Autodesk Fusion 360 part; units mm, degrees
(part 24 of 40)
  line L3969 (68.5452, -19.8469) -> (68.5908, -19.8966) construction
  line L3970 (68.5908, -19.8966) -> (68.6136, -19.9215) construction
  line L3971 (-51.1066, 30.2798) -> (-52.5103, 31.1115)
  line L3972 (54.5366, 23.5481) -> (56.0345, 24.1948)
  line L3973 (57.9623, 13.005) -> (59.5542, 13.3622)
  line L3974 (13.005, -57.9623) -> (13.3622, -59.5542)
  arc A98 (67.2191, -24.2132) -> (68.6136, -19.9215) centre (0, 0) ccw
  line L3975 (30.2798, 51.1066) -> (31.1115, 52.5103)
  spline S53 degree 5 poles (45.8153, 40.3263) (45.8385, 40.3467) (45.8854, 40.3868) (45.9573, 40.4451) (46.056, 40.5192) (46.1833, 40.6066) (46.3135, 40.6904) (46.4454, 40.772) (46.5782, 40.8524) (46.7117, 40.932) (46.8458, 41.0107) (46.9807, 41.0883) (47.1168, 41.1642) (47.2543, 41.2383) (47.393, 41.3106) (47.5329, 41.3813) (47.6738, 41.4504) (47.8156, 41.5184) (47.9581, 41.5853) (48.1012, 41.6512) (48.245, 41.716) (48.3895, 41.7798) (48.5347, 41.8424) (48.6807, 41.9039) (48.8274, 41.9642) (48.9749, 42.0234) (49.123, 42.0815) (49.2717, 42.1386) (49.421, 42.1947) (49.5709, 42.2499) (49.7214, 42.3041) (49.8724, 42.3574) (50.024, 42.4097) (50.1761, 42.461) (50.3288, 42.5114) (50.482, 42.5608) (50.6358, 42.6094) (50.79, 42.657) (50.9447, 42.7037) (51.0999, 42.7495) (51.2556, 42.7945) (51.4118, 42.8386) (51.5684, 42.8818) (51.7255, 42.9241) (51.883, 42.9656) (52.0409, 43.0063) (52.1993, 43.0461) (52.3581, 43.085) (52.5173, 43.1231) (52.6769, 43.1604) (52.8369, 43.1969) (52.9973, 43.2326) (53.1581, 43.2674) (53.3193, 43.3015) (53.4809, 43.3347) (53.6428, 43.3672) (53.8051, 43.3988) (53.9677, 43.4297) (54.1307, 43.4597) (54.294, 43.489) (54.4577, 43.5175) (54.6217, 43.5453) (54.7861, 43.5723) (54.9508, 43.5984) (55.1158, 43.6239) (55.2811, 43.6486) (55.4467, 43.6725) (55.6126, 43.6956) (55.7789, 43.718) (55.9454, 43.7397) (56.1122, 43.7606) (56.2459, 43.7767) (56.3463, 43.7885) (56.4133, 43.7962) (56.4469, 43.8) knots 0 0 0 0 0 0 0.01428571 0.02857143 0.04285714 0.05714286 0.07142857 0.08571429 0.1 0.11428571 0.12857143 0.14285714 0.15714286 0.17142857 0.18571429 0.2 0.21428571 0.22857143 0.24285714 0.25714286 0.27142857 0.28571429 0.3 0.31428571 0.32857143 0.34285714 0.35714286 0.37142857 0.38571429 0.4 0.41428571 0.42857143 0.44285714 0.45714286 0.47142857 0.48571429 0.5 0.51428571 0.52857143 0.54285714 0.55714286 0.57142857 0.58571429 0.6 0.61428571 0.62857143 0.64285714 0.65714286 0.67142857 0.68571429 0.7 0.71428571 0.72857143 0.74285714 0.75714286 0.77142857 0.78571429 0.8 0.81428571 0.82857143 0.84285714 0.85714286 0.87142857 0.88571429 0.9 0.91428571 0.92857143 0.94285714 0.95714286 0.97142857 0.98571429 1 1 1 1 1 1
  line L3976 (45.8153, 40.3263) -> (45.8385, 40.3467) construction
  line L3977 (45.8385, 40.3467) -> (45.8854, 40.3868) construction
  line L3978 (45.8854, 40.3868) -> (45.9573, 40.4451) construction
  line L3979 (45.9573, 40.4451) -> (46.056, 40.5192) construction
  line L3980 (46.056, 40.5192) -> (46.1833, 40.6066) construction
  line L3981 (46.1833, 40.6066) -> (46.3135, 40.6904) construction
  line L3982 (46.3135, 40.6904) -> (46.4454, 40.772) construction
  line L3983 (46.4454, 40.772) -> (46.5782, 40.8524) construction
  line L3984 (46.5782, 40.8524) -> (46.7117, 40.932) construction
  line L3985 (46.7117, 40.932) -> (46.8458, 41.0107) construction
  line L3986 (46.8458, 41.0107) -> (46.9807, 41.0883) construction
  line L3987 (46.9807, 41.0883) -> (47.1168, 41.1642) construction
  line L3988 (47.1168, 41.1642) -> (47.2543, 41.2383) construction
  line L3989 (47.2543, 41.2383) -> (47.393, 41.3106) construction
  line L3990 (47.393, 41.3106) -> (47.5329, 41.3813) construction
  line L3991 (47.5329, 41.3813) -> (47.6738, 41.4504) construction
  line L3992 (47.6738, 41.4504) -> (47.8156, 41.5184) construction
  line L3993 (47.8156, 41.5184) -> (47.9581, 41.5853) construction
  line L3994 (47.9581, 41.5853) -> (48.1012, 41.6512) construction
  line L3995 (48.1012, 41.6512) -> (48.245, 41.716) construction
  line L3996 (48.245, 41.716) -> (48.3895, 41.7798) construction
  line L3997 (48.3895, 41.7798) -> (48.5347, 41.8424) construction
  line L3998 (48.5347, 41.8424) -> (48.6807, 41.9039) construction
  line L3999 (48.6807, 41.9039) -> (48.8274, 41.9642) construction
  line L4000 (48.8274, 41.9642) -> (48.9749, 42.0234) construction
  line L4001 (48.9749, 42.0234) -> (49.123, 42.0815) construction
  line L4002 (49.123, 42.0815) -> (49.2717, 42.1386) construction
  line L4003 (49.2717, 42.1386) -> (49.421, 42.1947) construction
  line L4004 (49.421, 42.1947) -> (49.5709, 42.2499) construction
  line L4005 (49.5709, 42.2499) -> (49.7214, 42.3041) construction
  line L4006 (49.7214, 42.3041) -> (49.8724, 42.3574) construction
  line L4007 (49.8724, 42.3574) -> (50.024, 42.4097) construction
  line L4008 (50.024, 42.4097) -> (50.1761, 42.461) construction
  line L4009 (50.1761, 42.461) -> (50.3288, 42.5114) construction
  line L4010 (50.3288, 42.5114) -> (50.482, 42.5608) construction
  line L4011 (50.482, 42.5608) -> (50.6358, 42.6094) construction
  line L4012 (50.6358, 42.6094) -> (50.79, 42.657) construction
  line L4013 (50.79, 42.657) -> (50.9447, 42.7037) construction
  line L4014 (50.9447, 42.7037) -> (51.0999, 42.7495) construction
  line L4015 (51.0999, 42.7495) -> (51.2556, 42.7945) construction
  line L4016 (51.2556, 42.7945) -> (51.4118, 42.8386) construction
  line L4017 (51.4118, 42.8386) -> (51.5684, 42.8818) construction
  line L4018 (51.5684, 42.8818) -> (51.7255, 42.9241) construction
  line L4019 (51.7255, 42.9241) -> (51.883, 42.9656) construction
  line L4020 (51.883, 42.9656) -> (52.0409, 43.0063) construction
  line L4021 (52.0409, 43.0063) -> (52.1993, 43.0461) construction
  line L4022 (52.1993, 43.0461) -> (52.3581, 43.085) construction
  line L4023 (52.3581, 43.085) -> (52.5173, 43.1231) construction
  line L4024 (52.5173, 43.1231) -> (52.6769, 43.1604) construction
  line L4025 (52.6769, 43.1604) -> (52.8369, 43.1969) construction
  line L4026 (52.8369, 43.1969) -> (52.9973, 43.2326) construction
  line L4027 (52.9973, 43.2326) -> (53.1581, 43.2674) construction
  line L4028 (53.1581, 43.2674) -> (53.3193, 43.3015) construction
  line L4029 (53.3193, 43.3015) -> (53.4809, 43.3347) construction
  line L4030 (53.4809, 43.3347) -> (53.6428, 43.3672) construction
  line L4031 (53.6428, 43.3672) -> (53.8051, 43.3988) construction
  line L4032 (53.8051, 43.3988) -> (53.9677, 43.4297) construction
  line L4033 (53.9677, 43.4297) -> (54.1307, 43.4597) construction
  line L4034 (54.1307, 43.4597) -> (54.294, 43.489) construction
  line L4035 (54.294, 43.489) -> (54.4577, 43.5175) construction
  line L4036 (54.4577, 43.5175) -> (54.6217, 43.5453) construction
  line L4037 (54.6217, 43.5453) -> (54.7861, 43.5723) construction
  line L4038 (54.7861, 43.5723) -> (54.9508, 43.5984) construction
  line L4039 (54.9508, 43.5984) -> (55.1158, 43.6239) construction
  line L4040 (55.1158, 43.6239) -> (55.2811, 43.6486) construction
  line L4041 (55.2811, 43.6486) -> (55.4467, 43.6725) construction
  line L4042 (55.4467, 43.6725) -> (55.6126, 43.6956) construction
  line L4043 (55.6126, 43.6956) -> (55.7789, 43.718) construction
  line L4044 (55.7789, 43.718) -> (55.9454, 43.7397) construction
  line L4045 (55.9454, 43.7397) -> (56.1122, 43.7606) construction
  line L4046 (56.1122, 43.7606) -> (56.2459, 43.7767) construction
  line L4047 (56.2459, 43.7767) -> (56.3463, 43.7885) construction
  line L4048 (56.3463, 43.7885) -> (56.4133, 43.7962) construction
  line L4049 (56.4133, 43.7962) -> (56.4469, 43.8) construction
  arc A99 (7.2806, -56.9737) -> (5.5428, -59.1442) centre (7.5341, -58.9575) ccw
  arc A100 (27.5982, 50.3721) -> (24.5301, 51.9354) centre (0, 0) ccw
  arc A101 (-56.9737, -7.2806) -> (-59.1442, -5.5428) centre (-58.9575, -7.5341) ccw
  arc A102 (51.1066, 30.2798) -> (50.3721, 27.5982) centre (52.1261, 28.5592) ccw
  arc A103 (7.2806, -56.9737) -> (10.6816, -56.435) centre (0, 0) ccw
  arc A104 (-44.5906, 39.2483) -> (-41.8132, 39.3784) centre (-43.2692, 40.7496) ccw
  spline S54 degree 5 poles (-5.6951, -60.7685) (-5.6979, -60.7993) (-5.7029, -60.8609) (-5.7078, -60.9533) (-5.7097, -61.0766) (-5.7056, -61.231) (-5.6969, -61.3856) (-5.6854, -61.5403) (-5.6723, -61.695) (-5.6583, -61.8498) (-5.6431, -62.0045) (-5.6265, -62.1593) (-5.608, -62.314) (-5.5871, -62.4688) (-5.5641, -62.6235) (-5.539, -62.7782) (-5.5121, -62.9329) (-5.4838, -63.0875) (-5.4542, -63.2421) (-5.4233, -63.3966) (-5.3913, -63.5511) (-5.3579, -63.7055) (-5.3232, -63.8598) (-5.2871, -64.014) (-5.2497, -64.1682) (-5.2109, -64.3222) (-5.1709, -64.4762) (-5.1297, -64.6301) (-5.0873, -64.7839) (-5.0439, -64.9376) (-4.9993, -65.0912) (-4.9536, -65.2447) (-4.9068, -65.398) (-4.8589, -65.5513) (-4.8099, -65.7044) (-4.7599, -65.8574) (-4.7087, -66.0103) (-4.6566, -66.1631) (-4.6035, -66.3158) (-4.5493, -66.4683) (-4.4942, -66.6206) (-4.438, -66.7729) (-4.381, -66.925) (-4.3229, -67.077) (-4.2639, -67.2288) (-4.2039, -67.3804) (-4.143, -67.532) (-4.0812, -67.6833) (-4.0185, -67.8345) (-3.9548, -67.9856) (-3.8903, -68.1365) (-3.8249, -68.2872) (-3.7585, -68.4378) (-3.6913, -68.5882) (-3.6233, -68.7384) (-3.5543, -68.8885) (-3.4846, -69.0384) (-3.4139, -69.1881) (-3.3425, -69.3376) (-3.2701, -69.487) (-3.197, -69.6362) (-3.123, -69.7852) (-3.0482, -69.934) (-2.9726, -70.0826) (-2.8962, -70.2311) (-2.819, -70.3793) (-2.741, -70.5274) (-2.6622, -70.6752) (-2.5826, -70.8229) (-2.5023, -70.9703) (-2.4211, -71.1176) (-2.3556, -71.2352) (-2.3061, -71.3234) (-2.2729, -71.3821) (-2.2563, -71.4115) knots 0 0 0 0 0 0 0.01428571 0.02857143 0.04285714 0.05714286 0.07142857 0.08571429 0.1 0.11428571 0.12857143 0.14285714 0.15714286 0.17142857 0.18571429 0.2 0.21428571 0.22857143 0.24285714 0.25714286 0.27142857 0.28571429 0.3 0.31428571 0.32857143 0.34285714 0.35714286 0.37142857 0.38571429 0.4 0.41428571 0.42857143 0.44285714 0.45714286 0.47142857 0.48571429 0.5 0.51428571 0.52857143 0.54285714 0.55714286 0.57142857 0.58571429 0.6 0.61428571 0.62857143 0.64285714 0.65714286 0.67142857 0.68571429 0.7 0.71428571 0.72857143 0.74285714 0.75714286 0.77142857 0.78571429 0.8 0.81428571 0.82857143 0.84285714 0.85714286 0.87142857 0.88571429 0.9 0.91428571 0.92857143 0.94285714 0.95714286 0.97142857 0.98571429 1 1 1 1 1 1
  line L4050 (-5.6951, -60.7685) -> (-5.6979, -60.7993) construction
  line L4051 (-5.6979, -60.7993) -> (-5.7029, -60.8609) construction
  line L4052 (-5.7029, -60.8609) -> (-5.7078, -60.9533) construction
  line L4053 (-5.7078, -60.9533) -> (-5.7097, -61.0766) construction
  line L4054 (-5.7097, -61.0766) -> (-5.7056, -61.231) construction
  line L4055 (-5.7056, -61.231) -> (-5.6969, -61.3856) construction
  line L4056 (-5.6969, -61.3856) -> (-5.6854, -61.5403) construction
  line L4057 (-5.6854, -61.5403) -> (-5.6723, -61.695) construction
  line L4058 (-5.6723, -61.695) -> (-5.6583, -61.8498) construction
  line L4059 (-5.6583, -61.8498) -> (-5.6431, -62.0045) construction
  line L4060 (-5.6431, -62.0045) -> (-5.6265, -62.1593) construction
  line L4061 (-5.6265, -62.1593) -> (-5.608, -62.314) construction
  line L4062 (-5.608, -62.314) -> (-5.5871, -62.4688) construction
  line L4063 (-5.5871, -62.4688) -> (-5.5641, -62.6235) construction
  line L4064 (-5.5641, -62.6235) -> (-5.539, -62.7782) construction
  line L4065 (-5.539, -62.7782) -> (-5.5121, -62.9329) construction
  line L4066 (-5.5121, -62.9329) -> (-5.4838, -63.0875) construction
  line L4067 (-5.4838, -63.0875) -> (-5.4542, -63.2421) construction
  line L4068 (-5.4542, -63.2421) -> (-5.4233, -63.3966) construction
  line L4069 (-5.4233, -63.3966) -> (-5.3913, -63.5511) construction
  line L4070 (-5.3913, -63.5511) -> (-5.3579, -63.7055) construction
  line L4071 (-5.3579, -63.7055) -> (-5.3232, -63.8598) construction
  line L4072 (-5.3232, -63.8598) -> (-5.2871, -64.014) construction
  line L4073 (-5.2871, -64.014) -> (-5.2497, -64.1682) construction
  line L4074 (-5.2497, -64.1682) -> (-5.2109, -64.3222) construction
  line L4075 (-5.2109, -64.3222) -> (-5.1709, -64.4762) construction
  line L4076 (-5.1709, -64.4762) -> (-5.1297, -64.6301) construction
  line L4077 (-5.1297, -64.6301) -> (-5.0873, -64.7839) construction
  line L4078 (-5.0873, -64.7839) -> (-5.0439, -64.9376) construction
  line L4079 (-5.0439, -64.9376) -> (-4.9993, -65.0912) construction
  line L4080 (-4.9993, -65.0912) -> (-4.9536, -65.2447) construction
  line L4081 (-4.9536, -65.2447) -> (-4.9068, -65.398) construction
  line L4082 (-4.9068, -65.398) -> (-4.8589, -65.5513) construction
  line L4083 (-4.8589, -65.5513) -> (-4.8099, -65.7044) construction
  line L4084 (-4.8099, -65.7044) -> (-4.7599, -65.8574) construction
  line L4085 (-4.7599, -65.8574) -> (-4.7087, -66.0103) construction
  line L4086 (-4.7087, -66.0103) -> (-4.6566, -66.1631) construction
  line L4087 (-4.6566, -66.1631) -> (-4.6035, -66.3158) construction
  line L4088 (-4.6035, -66.3158) -> (-4.5493, -66.4683) construction
  line L4089 (-4.5493, -66.4683) -> (-4.4942, -66.6206) construction
  line L4090 (-4.4942, -66.6206) -> (-4.438, -66.7729) construction
  line L4091 (-4.438, -66.7729) -> (-4.381, -66.925) construction
  line L4092 (-4.381, -66.925) -> (-4.3229, -67.077) construction
  line L4093 (-4.3229, -67.077) -> (-4.2639, -67.2288) construction
  line L4094 (-4.2639, -67.2288) -> (-4.2039, -67.3804) construction
  line L4095 (-4.2039, -67.3804) -> (-4.143, -67.532) construction
  line L4096 (-4.143, -67.532) -> (-4.0812, -67.6833) construction
  line L4097 (-4.0812, -67.6833) -> (-4.0185, -67.8345) construction
  line L4098 (-4.0185, -67.8345) -> (-3.9548, -67.9856) construction
  line L4099 (-3.9548, -67.9856) -> (-3.8903, -68.1365) construction
  line L4100 (-3.8903, -68.1365) -> (-3.8249, -68.2872) construction
  line L4101 (-3.8249, -68.2872) -> (-3.7585, -68.4378) construction
  line L4102 (-3.7585, -68.4378) -> (-3.6913, -68.5882) construction
  line L4103 (-3.6913, -68.5882) -> (-3.6233, -68.7384) construction
  line L4104 (-3.6233, -68.7384) -> (-3.5543, -68.8885) construction
  line L4105 (-3.5543, -68.8885) -> (-3.4846, -69.0384) construction
  line L4106 (-3.4846, -69.0384) -> (-3.4139, -69.1881) construction
  line L4107 (-3.4139, -69.1881) -> (-3.3425, -69.3376) construction
  line L4108 (-3.3425, -69.3376) -> (-3.2701, -69.487) construction
  line L4109 (-3.2701, -69.487) -> (-3.197, -69.6362) construction
  line L4110 (-3.197, -69.6362) -> (-3.123, -69.7852) construction
  line L4111 (-3.123, -69.7852) -> (-3.0482, -69.934) construction
  line L4112 (-3.0482, -69.934) -> (-2.9726, -70.0826) construction
  line L4113 (-2.9726, -70.0826) -> (-2.8962, -70.2311) construction
  line L4114 (-2.8962, -70.2311) -> (-2.819, -70.3793) construction
  line L4115 (-2.819, -70.3793) -> (-2.741, -70.5274) construction
  line L4116 (-2.741, -70.5274) -> (-2.6622, -70.6752) construction
  line L4117 (-2.6622, -70.6752) -> (-2.5826, -70.8229) construction
  line L4118 (-2.5826, -70.8229) -> (-2.5023, -70.9703) construction
  line L4119 (-2.5023, -70.9703) -> (-2.4211, -71.1176) construction
  line L4120 (-2.4211, -71.1176) -> (-2.3556, -71.2352) construction
  line L4121 (-2.3556, -71.2352) -> (-2.3061, -71.3234) construction
  line L4122 (-2.3061, -71.3234) -> (-2.2729, -71.3821) construction
  line L4123 (-2.2729, -71.3821) -> (-2.2563, -71.4115) construction
  spline S55 degree 5 poles (31.1115, -52.5103) (31.1272, -52.5368) (31.1594, -52.5895) (31.2097, -52.6672) (31.2807, -52.7681) (31.3748, -52.8906) (31.4727, -53.0106) (31.5729, -53.1289) (31.6744, -53.2464) (31.7767, -53.3634) (31.88, -53.4797) (31.9844, -53.5951) (32.0903, -53.7094) (32.1981, -53.8224) (32.3077, -53.934) (32.419, -54.0444) (32.5316, -54.1537) (32.6455, -54.2622) (32.7603, -54.3698) (32.876, -54.4767) (32.9927, -54.5828) (33.1105, -54.6881) (33.2292, -54.7926) (33.3491, -54.8961) (33.47, -54.9988) (33.5919, -55.1007) (33.7148, -55.2017) (33.8386, -55.302) (33.9633, -55.4015) (34.0888, -55.5003) (34.2151, -55.5984) (34.3423, -55.6957) (34.4703, -55.7923) (34.5991, -55.8881) (34.7288, -55.9832) (34.8592, -56.0776) (34.9905, -56.1712) (35.1224, -56.2642) (35.2552, -56.3564) (35.3886, -56.448) (35.5228, -56.5388) (35.6577, -56.629) (35.7933, -56.7185) (35.9295, -56.8073) (36.0665, -56.8955) (36.2042, -56.9829) (36.3425, -57.0697) (36.4815, -57.1558) (36.6211, -57.2413) (36.7614, -57.3261) (36.9023, -57.4102) (37.0438, -57.4937) (37.186, -57.5765) (37.3288, -57.6587) (37.4721, -57.7403) (37.6161, -57.8212) (37.7607, -57.9014) (37.9058, -57.981) (38.0515, -58.06) (38.1978, -58.1383) (38.3447, -58.216) (38.4921, -58.2931) (38.6401, -58.3695) (38.7886, -58.4453) (38.9377, -58.5205) (39.0873, -58.595) (39.2374, -58.669) (39.3881, -58.7423) (39.5393, -58.8149) (39.6909, -58.887) (39.8431, -58.9584) (39.9653, -59.0151) (40.0572, -59.0573) (40.1185, -59.0853) (40.1492, -59.0993) knots 0 0 0 0 0 0 0.01428571 0.02857143 0.04285714 0.05714286 0.07142857 0.08571429 0.1 0.11428571 0.12857143 0.14285714 0.15714286 0.17142857 0.18571429 0.2 0.21428571 0.22857143 0.24285714 0.25714286 0.27142857 0.28571429 0.3 0.31428571 0.32857143 0.34285714 0.35714286 0.37142857 0.38571429 0.4 0.41428571 0.42857143 0.44285714 0.45714286 0.47142857 0.48571429 0.5 0.51428571 0.52857143 0.54285714 0.55714286 0.57142857 0.58571429 0.6 0.61428571 0.62857143 0.64285714 0.65714286 0.67142857 0.68571429 0.7 0.71428571 0.72857143 0.74285714 0.75714286 0.77142857 0.78571429 0.8 0.81428571 0.82857143 0.84285714 0.85714286 0.87142857 0.88571429 0.9 0.91428571 0.92857143 0.94285714 0.95714286 0.97142857 0.98571429 1 1 1 1 1 1
  line L4124 (31.1115, -52.5103) -> (31.1272, -52.5368) construction
  line L4125 (31.1272, -52.5368) -> (31.1594, -52.5895) construction
  line L4126 (31.1594, -52.5895) -> (31.2097, -52.6672) construction
  line L4127 (31.2097, -52.6672) -> (31.2807, -52.7681) construction
  line L4128 (31.2807, -52.7681) -> (31.3748, -52.8906) construction
  line L4129 (31.3748, -52.8906) -> (31.4727, -53.0106) construction
  line L4130 (31.4727, -53.0106) -> (31.5729, -53.1289) construction
  line L4131 (31.5729, -53.1289) -> (31.6744, -53.2464) construction
  line L4132 (31.6744, -53.2464) -> (31.7767, -53.3634) construction
  line L4133 (31.7767, -53.3634) -> (31.88, -53.4797) construction
  line L4134 (31.88, -53.4797) -> (31.9844, -53.5951) construction
  line L4135 (31.9844, -53.5951) -> (32.0903, -53.7094) construction
  line L4136 (32.0903, -53.7094) -> (32.1981, -53.8224) construction
  line L4137 (32.1981, -53.8224) -> (32.3077, -53.934) construction
  line L4138 (32.3077, -53.934) -> (32.419, -54.0444) construction
  line L4139 (32.419, -54.0444) -> (32.5316, -54.1537) construction
  line L4140 (32.5316, -54.1537) -> (32.6455, -54.2622) construction
  line L4141 (32.6455, -54.2622) -> (32.7603, -54.3698) construction
  line L4142 (32.7603, -54.3698) -> (32.876, -54.4767) construction
  line L4143 (32.876, -54.4767) -> (32.9927, -54.5828) construction
  line L4144 (32.9927, -54.5828) -> (33.1105, -54.6881) construction
  line L4145 (33.1105, -54.6881) -> (33.2292, -54.7926) construction
  line L4146 (33.2292, -54.7926) -> (33.3491, -54.8961) construction
  line L4147 (33.3491, -54.8961) -> (33.47, -54.9988) construction
  line L4148 (33.47, -54.9988) -> (33.5919, -55.1007) construction
  line L4149 (33.5919, -55.1007) -> (33.7148, -55.2017) construction
  line L4150 (33.7148, -55.2017) -> (33.8386, -55.302) construction
  line L4151 (33.8386, -55.302) -> (33.9633, -55.4015) construction
  line L4152 (33.9633, -55.4015) -> (34.0888, -55.5003) construction
  line L4153 (34.0888, -55.5003) -> (34.2151, -55.5984) construction
  line L4154 (34.2151, -55.5984) -> (34.3423, -55.6957) construction
  line L4155 (34.3423, -55.6957) -> (34.4703, -55.7923) construction
  line L4156 (34.4703, -55.7923) -> (34.5991, -55.8881) construction
  line L4157 (34.5991, -55.8881) -> (34.7288, -55.9832) construction
  line L4158 (34.7288, -55.9832) -> (34.8592, -56.0776) construction
  line L4159 (34.8592, -56.0776) -> (34.9905, -56.1712) construction
  line L4160 (34.9905, -56.1712) -> (35.1224, -56.2642) construction
  line L4161 (35.1224, -56.2642) -> (35.2552, -56.3564) construction
  line L4162 (35.2552, -56.3564) -> (35.3886, -56.448) construction
  line L4163 (35.3886, -56.448) -> (35.5228, -56.5388) construction
  line L4164 (35.5228, -56.5388) -> (35.6577, -56.629) construction
  line L4165 (35.6577, -56.629) -> (35.7933, -56.7185) construction
  line L4166 (35.7933, -56.7185) -> (35.9295, -56.8073) construction
  line L4167 (35.9295, -56.8073) -> (36.0665, -56.8955) construction
  line L4168 (36.0665, -56.8955) -> (36.2042, -56.9829) construction
  line L4169 (36.2042, -56.9829) -> (36.3425, -57.0697) construction
  line L4170 (36.3425, -57.0697) -> (36.4815, -57.1558) construction
  line L4171 (36.4815, -57.1558) -> (36.6211, -57.2413) construction
  line L4172 (36.6211, -57.2413) -> (36.7614, -57.3261) construction
  line L4173 (36.7614, -57.3261) -> (36.9023, -57.4102) construction
  line L4174 (36.9023, -57.4102) -> (37.0438, -57.4937) construction
  line L4175 (37.0438, -57.4937) -> (37.186, -57.5765) construction
  line L4176 (37.186, -57.5765) -> (37.3288, -57.6587) construction
  line L4177 (37.3288, -57.6587) -> (37.4721, -57.7403) construction
  line L4178 (37.4721, -57.7403) -> (37.6161, -57.8212) construction
  line L4179 (37.6161, -57.8212) -> (37.7607, -57.9014) construction
  line L4180 (37.7607, -57.9014) -> (37.9058, -57.981) construction
  line L4181 (37.9058, -57.981) -> (38.0515, -58.06) construction
  line L4182 (38.0515, -58.06) -> (38.1978, -58.1383) construction
  line L4183 (38.1978, -58.1383) -> (38.3447, -58.216) construction
  line L4184 (38.3447, -58.216) -> (38.4921, -58.2931) construction
  line L4185 (38.4921, -58.2931) -> (38.6401, -58.3695) construction
  line L4186 (38.6401, -58.3695) -> (38.7886, -58.4453) construction
  line L4187 (38.7886, -58.4453) -> (38.9377, -58.5205) construction
  line L4188 (38.9377, -58.5205) -> (39.0873, -58.595) construction
  line L4189 (39.0873, -58.595) -> (39.2374, -58.669) construction
  line L4190 (39.2374, -58.669) -> (39.3881, -58.7423) construction
  line L4191 (39.3881, -58.7423) -> (39.5393, -58.8149) construction
  line L4192 (39.5393, -58.8149) -> (39.6909, -58.887) construction
  line L4193 (39.6909, -58.887) -> (39.8431, -58.9584) construction
  line L4194 (39.8431, -58.9584) -> (39.9653, -59.0151) construction
  line L4195 (39.9653, -59.0151) -> (40.0572, -59.0573) construction
  line L4196 (40.0572, -59.0573) -> (40.1185, -59.0853) construction
  line L4197 (40.1185, -59.0853) -> (40.1492, -59.0993) construction
  line L4198 (-30.2798, -51.1066) -> (-31.1115, -52.5103)
  line L4199 (-39.2483, 44.5906) -> (-40.3263, 45.8153)
  arc A105 (-7.2806, 56.9737) -> (-5.5428, 59.1442) centre (-7.5341, 58.9575) ccw
  line L4200 (23.5481, -54.5366) -> (24.1948, -56.0345)
  arc A106 (56.9737, 7.2806) -> (56.435, 10.6816) centre (0, 0) ccw
  arc A107 (-10.6816, -56.435) -> (-7.2806, -56.9737) centre (0, 0) ccw
  spline S56 degree 5 poles (-13.3622, 59.5542) (-13.369, 59.5843) (-13.3833, 59.6444) (-13.4071, 59.7338) (-13.4435, 59.8517) (-13.4951, 59.9973) (-13.5511, 60.1416) (-13.6099, 60.2852) (-13.6701, 60.4283) (-13.7313, 60.5711) (-13.7935, 60.7136) (-13.8571, 60.8557) (-13.9226, 60.9971) (-13.9902, 61.1379) (-14.06, 61.2779) (-14.1316, 61.4173) (-14.205, 61.5561) (-14.2797, 61.6944) (-14.3557, 61.8322) (-14.4327, 61.9697) (-14.5109, 62.1067) (-14.5904, 62.2432) (-14.6711, 62.3792) (-14.753, 62.5148) (-14.8363, 62.6498) (-14.9208, 62.7843) (-15.0064, 62.9184) (-15.0932, 63.052) (-15.181, 63.1852) (-15.2698, 63.318) (-15.3597, 63.4503) (-15.4506, 63.5821) (-15.5425, 63.7135) (-15.6354, 63.8445) (-15.7293, 63.975) (-15.8242, 64.105) (-15.92, 64.2346) (-16.0168, 64.3638) (-16.1146, 64.4926) (-16.2132, 64.6209) (-16.3127, 64.7488) (-16.4131, 64.8762) (-16.5144, 65.0032) (-16.6166, 65.1298) (-16.7196, 65.256) (-16.8235, 65.3817) (-16.9283, 65.507) (-17.0338, 65.6318) (-17.1402, 65.7562) (-17.2474, 65.8802) (-17.3555, 66.0038) (-17.4643, 66.1269) (-17.5739, 66.2497) (-17.6842, 66.3719) (-17.7954, 66.4938) (-17.9073, 66.6152) (-18.02, 66.7362) (-18.1335, 66.8568) (-18.2477, 66.9769) (-18.3626, 67.0966) (-18.4782, 67.2159) (-18.5946, 67.3347) (-18.7118, 67.4531) (-18.8296, 67.5711) (-18.9481, 67.6887) (-19.0674, 67.8058) (-19.1873, 67.9225) (-19.3079, 68.0388) (-19.4293, 68.1546) (-19.5512, 68.27) (-19.6739, 68.385) (-19.7726, 68.4767) (-19.8469, 68.5452) (-19.8966, 68.5908) (-19.9215, 68.6136) knots 0 0 0 0 0 0 0.01428571 0.02857143 0.04285714 0.05714286 0.07142857 0.08571429 0.1 0.11428571 0.12857143 0.14285714 0.15714286 0.17142857 0.18571429 0.2 0.21428571 0.22857143 0.24285714 0.25714286 0.27142857 0.28571429 0.3 0.31428571 0.32857143 0.34285714 0.35714286 0.37142857 0.38571429 0.4 0.41428571 0.42857143 0.44285714 0.45714286 0.47142857 0.48571429 0.5 0.51428571 0.52857143 0.54285714 0.55714286 0.57142857 0.58571429 0.6 0.61428571 0.62857143 0.64285714 0.65714286 0.67142857 0.68571429 0.7 0.71428571 0.72857143 0.74285714 0.75714286 0.77142857 0.78571429 0.8 0.81428571 0.82857143 0.84285714 0.85714286 0.87142857 0.88571429 0.9 0.91428571 0.92857143 0.94285714 0.95714286 0.97142857 0.98571429 1 1 1 1 1 1
  line L4201 (-13.3622, 59.5542) -> (-13.369, 59.5843) construction
  line L4202 (-13.369, 59.5843) -> (-13.3833, 59.6444) construction
  line L4203 (-13.3833, 59.6444) -> (-13.4071, 59.7338) construction
  line L4204 (-13.4071, 59.7338) -> (-13.4435, 59.8517) construction
  line L4205 (-13.4435, 59.8517) -> (-13.4951, 59.9973) construction
  line L4206 (-13.4951, 59.9973) -> (-13.5511, 60.1416) construction
  line L4207 (-13.5511, 60.1416) -> (-13.6099, 60.2852) construction
  line L4208 (-13.6099, 60.2852) -> (-13.6701, 60.4283) construction
  line L4209 (-13.6701, 60.4283) -> (-13.7313, 60.5711) construction
  line L4210 (-13.7313, 60.5711) -> (-13.7935, 60.7136) construction
  line L4211 (-13.7935, 60.7136) -> (-13.8571, 60.8557) construction
  line L4212 (-13.8571, 60.8557) -> (-13.9226, 60.9971) construction
  line L4213 (-13.9226, 60.9971) -> (-13.9902, 61.1379) construction
  line L4214 (-13.9902, 61.1379) -> (-14.06, 61.2779) construction
  line L4215 (-14.06, 61.2779) -> (-14.1316, 61.4173) construction
  line L4216 (-14.1316, 61.4173) -> (-14.205, 61.5561) construction
  line L4217 (-14.205, 61.5561) -> (-14.2797, 61.6944) construction
  line L4218 (-14.2797, 61.6944) -> (-14.3557, 61.8322) construction
  line L4219 (-14.3557, 61.8322) -> (-14.4327, 61.9697) construction
  line L4220 (-14.4327, 61.9697) -> (-14.5109, 62.1067) construction
  line L4221 (-14.5109, 62.1067) -> (-14.5904, 62.2432) construction
  line L4222 (-14.5904, 62.2432) -> (-14.6711, 62.3792) construction
  line L4223 (-14.6711, 62.3792) -> (-14.753, 62.5148) construction
  line L4224 (-14.753, 62.5148) -> (-14.8363, 62.6498) construction
  line L4225 (-14.8363, 62.6498) -> (-14.9208, 62.7843) construction
  line L4226 (-14.9208, 62.7843) -> (-15.0064, 62.9184) construction
  line L4227 (-15.0064, 62.9184) -> (-15.0932, 63.052) construction
  line L4228 (-15.0932, 63.052) -> (-15.181, 63.1852) construction
  line L4229 (-15.181, 63.1852) -> (-15.2698, 63.318) construction
  line L4230 (-15.2698, 63.318) -> (-15.3597, 63.4503) construction
  line L4231 (-15.3597, 63.4503) -> (-15.4506, 63.5821) construction
  line L4232 (-15.4506, 63.5821) -> (-15.5425, 63.7135) construction
  line L4233 (-15.5425, 63.7135) -> (-15.6354, 63.8445) construction
  line L4234 (-15.6354, 63.8445) -> (-15.7293, 63.975) construction
  line L4235 (-15.7293, 63.975) -> (-15.8242, 64.105) construction
  line L4236 (-15.8242, 64.105) -> (-15.92, 64.2346) construction
  line L4237 (-15.92, 64.2346) -> (-16.0168, 64.3638) construction
  line L4238 (-16.0168, 64.3638) -> (-16.1146, 64.4926) construction
  line L4239 (-16.1146, 64.4926) -> (-16.2132, 64.6209) construction
  line L4240 (-16.2132, 64.6209) -> (-16.3127, 64.7488) construction
  line L4241 (-16.3127, 64.7488) -> (-16.4131, 64.8762) construction
  line L4242 (-16.4131, 64.8762) -> (-16.5144, 65.0032) construction
  line L4243 (-16.5144, 65.0032) -> (-16.6166, 65.1298) construction
  line L4244 (-16.6166, 65.1298) -> (-16.7196, 65.256) construction
  line L4245 (-16.7196, 65.256) -> (-16.8235, 65.3817) construction
  line L4246 (-16.8235, 65.3817) -> (-16.9283, 65.507) construction
  line L4247 (-16.9283, 65.507) -> (-17.0338, 65.6318) construction
  line L4248 (-17.0338, 65.6318) -> (-17.1402, 65.7562) construction
  line L4249 (-17.1402, 65.7562) -> (-17.2474, 65.8802) construction
  line L4250 (-17.2474, 65.8802) -> (-17.3555, 66.0038) construction
  line L4251 (-17.3555, 66.0038) -> (-17.4643, 66.1269) construction
  line L4252 (-17.4643, 66.1269) -> (-17.5739, 66.2497) construction
  line L4253 (-17.5739, 66.2497) -> (-17.6842, 66.3719) construction
  line L4254 (-17.6842, 66.3719) -> (-17.7954, 66.4938) construction
  line L4255 (-17.7954, 66.4938) -> (-17.9073, 66.6152) construction
  line L4256 (-17.9073, 66.6152) -> (-18.02, 66.7362) construction
  line L4257 (-18.02, 66.7362) -> (-18.1335, 66.8568) construction
  line L4258 (-18.1335, 66.8568) -> (-18.2477, 66.9769) construction
  line L4259 (-18.2477, 66.9769) -> (-18.3626, 67.0966) construction
  line L4260 (-18.3626, 67.0966) -> (-18.4782, 67.2159) construction
  line L4261 (-18.4782, 67.2159) -> (-18.5946, 67.3347) construction
  line L4262 (-18.5946, 67.3347) -> (-18.7118, 67.4531) construction
  line L4263 (-18.7118, 67.4531) -> (-18.8296, 67.5711) construction
  line L4264 (-18.8296, 67.5711) -> (-18.9481, 67.6887) construction
  line L4265 (-18.9481, 67.6887) -> (-19.0674, 67.8058) construction
  line L4266 (-19.0674, 67.8058) -> (-19.1873, 67.9225) construction
  line L4267 (-19.1873, 67.9225) -> (-19.3079, 68.0388) construction
  line L4268 (-19.3079, 68.0388) -> (-19.4293, 68.1546) construction
  line L4269 (-19.4293, 68.1546) -> (-19.5512, 68.27) construction
  line L4270 (-19.5512, 68.27) -> (-19.6739, 68.385) construction
  line L4271 (-19.6739, 68.385) -> (-19.7726, 68.4767) construction
  line L4272 (-19.7726, 68.4767) -> (-19.8469, 68.5452) construction
  line L4273 (-19.8469, 68.5452) -> (-19.8966, 68.5908) construction
  line L4274 (-19.8966, 68.5908) -> (-19.9215, 68.6136) construction
  arc A108 (-56.4469, 43.8) -> (-59.0993, 40.1492) centre (0, 0) ccw
  spline S57 degree 5 poles (-60.7685, -5.6951) (-60.7993, -5.6979) (-60.8609, -5.7029) (-60.9533, -5.7078) (-61.0766, -5.7097) (-61.231, -5.7056) (-61.3856, -5.6969) (-61.5403, -5.6854) (-61.695, -5.6723) (-61.8498, -5.6583) (-62.0045, -5.6431) (-62.1593, -5.6265) (-62.314, -5.608) (-62.4688, -5.5871) (-62.6235, -5.5641) (-62.7782, -5.539) (-62.9329, -5.5121) (-63.0875, -5.4838) (-63.2421, -5.4542) (-63.3966, -5.4233) (-63.5511, -5.3913) (-63.7055, -5.3579) (-63.8598, -5.3232) (-64.014, -5.2871) (-64.1682, -5.2497) (-64.3222, -5.2109) (-64.4762, -5.1709) (-64.6301, -5.1297) (-64.7839, -5.0873) (-64.9376, -5.0439) (-65.0912, -4.9993) (-65.2447, -4.9536) (-65.398, -4.9068) (-65.5513, -4.8589) (-65.7044, -4.8099) (-65.8574, -4.7599) (-66.0103, -4.7087) (-66.1631, -4.6566) (-66.3158, -4.6035) (-66.4683, -4.5493) (-66.6206, -4.4942) (-66.7729, -4.438) (-66.925, -4.381) (-67.077, -4.3229) (-67.2288, -4.2639) (-67.3804, -4.2039) (-67.532, -4.143) (-67.6833, -4.0812) (-67.8345, -4.0185) (-67.9856, -3.9548) (-68.1365, -3.8903) (-68.2872, -3.8249) (-68.4378, -3.7585) (-68.5882, -3.6913) (-68.7384, -3.6233) (-68.8885, -3.5543) (-69.0384, -3.4846) (-69.1881, -3.4139) (-69.3376, -3.3425) (-69.487, -3.2701) (-69.6362, -3.197) (-69.7852, -3.123) (-69.934, -3.0482) (-70.0826, -2.9726) (-70.2311, -2.8962) (-70.3793, -2.819) (-70.5274, -2.741) (-70.6752, -2.6622) (-70.8229, -2.5826) (-70.9703, -2.5023) (-71.1176, -2.4211) (-71.2352, -2.3556) (-71.3234, -2.3061) (-71.3821, -2.2729) (-71.4115, -2.2563) knots 0 0 0 0 0 0 0.01428571 0.02857143 0.04285714 0.05714286 0.07142857 0.08571429 0.1 0.11428571 0.12857143 0.14285714 0.15714286 0.17142857 0.18571429 0.2 0.21428571 0.22857143 0.24285714 0.25714286 0.27142857 0.28571429 0.3 0.31428571 0.32857143 0.34285714 0.35714286 0.37142857 0.38571429 0.4 0.41428571 0.42857143 0.44285714 0.45714286 0.47142857 0.48571429 0.5 0.51428571 0.52857143 0.54285714 0.55714286 0.57142857 0.58571429 0.6 0.61428571 0.62857143 0.64285714 0.65714286 0.67142857 0.68571429 0.7 0.71428571 0.72857143 0.74285714 0.75714286 0.77142857 0.78571429 0.8 0.81428571 0.82857143 0.84285714 0.85714286 0.87142857 0.88571429 0.9 0.91428571 0.92857143 0.94285714 0.95714286 0.97142857 0.98571429 1 1 1 1 1 1
  line L4275 (-60.7685, -5.6951) -> (-60.7993, -5.6979) construction
  line L4276 (-60.7993, -5.6979) -> (-60.8609, -5.7029) construction
  line L4277 (-60.8609, -5.7029) -> (-60.9533, -5.7078) construction
  line L4278 (-60.9533, -5.7078) -> (-61.0766, -5.7097) construction
  line L4279 (-61.0766, -5.7097) -> (-61.231, -5.7056) construction
  line L4280 (-61.231, -5.7056) -> (-61.3856, -5.6969) construction
  line L4281 (-61.3856, -5.6969) -> (-61.5403, -5.6854) construction
  line L4282 (-61.5403, -5.6854) -> (-61.695, -5.6723) construction
  line L4283 (-61.695, -5.6723) -> (-61.8498, -5.6583) construction
  line L4284 (-61.8498, -5.6583) -> (-62.0045, -5.6431) construction
  line L4285 (-62.0045, -5.6431) -> (-62.1593, -5.6265) construction
  line L4286 (-62.1593, -5.6265) -> (-62.314, -5.608) construction
  line L4287 (-62.314, -5.608) -> (-62.4688, -5.5871) construction
  line L4288 (-62.4688, -5.5871) -> (-62.6235, -5.5641) construction
  line L4289 (-62.6235, -5.5641) -> (-62.7782, -5.539) construction
  line L4290 (-62.7782, -5.539) -> (-62.9329, -5.5121) construction
  line L4291 (-62.9329, -5.5121) -> (-63.0875, -5.4838) construction
  line L4292 (-63.0875, -5.4838) -> (-63.2421, -5.4542) construction
  line L4293 (-63.2421, -5.4542) -> (-63.3966, -5.4233) construction
  line L4294 (-63.3966, -5.4233) -> (-63.5511, -5.3913) construction
  line L4295 (-63.5511, -5.3913) -> (-63.7055, -5.3579) construction
  line L4296 (-63.7055, -5.3579) -> (-63.8598, -5.3232) construction
  line L4297 (-63.8598, -5.3232) -> (-64.014, -5.2871) construction
  line L4298 (-64.014, -5.2871) -> (-64.1682, -5.2497) construction
  line L4299 (-64.1682, -5.2497) -> (-64.3222, -5.2109) construction
  line L4300 (-64.3222, -5.2109) -> (-64.4762, -5.1709) construction
  line L4301 (-64.4762, -5.1709) -> (-64.6301, -5.1297) construction
  line L4302 (-64.6301, -5.1297) -> (-64.7839, -5.0873) construction
  line L4303 (-64.7839, -5.0873) -> (-64.9376, -5.0439) construction
  line L4304 (-64.9376, -5.0439) -> (-65.0912, -4.9993) construction
  line L4305 (-65.0912, -4.9993) -> (-65.2447, -4.9536) construction
  line L4306 (-65.2447, -4.9536) -> (-65.398, -4.9068) construction
  line L4307 (-65.398, -4.9068) -> (-65.5513, -4.8589) construction
  line L4308 (-65.5513, -4.8589) -> (-65.7044, -4.8099) construction
  line L4309 (-65.7044, -4.8099) -> (-65.8574, -4.7599) construction
  line L4310 (-65.8574, -4.7599) -> (-66.0103, -4.7087) construction
  line L4311 (-66.0103, -4.7087) -> (-66.1631, -4.6566) construction
  line L4312 (-66.1631, -4.6566) -> (-66.3158, -4.6035) construction
  line L4313 (-66.3158, -4.6035) -> (-66.4683, -4.5493) construction
  line L4314 (-66.4683, -4.5493) -> (-66.6206, -4.4942) construction
  line L4315 (-66.6206, -4.4942) -> (-66.7729, -4.438) construction
  line L4316 (-66.7729, -4.438) -> (-66.925, -4.381) construction
  line L4317 (-66.925, -4.381) -> (-67.077, -4.3229) construction
  line L4318 (-67.077, -4.3229) -> (-67.2288, -4.2639) construction
  line L4319 (-67.2288, -4.2639) -> (-67.3804, -4.2039) construction
  line L4320 (-67.3804, -4.2039) -> (-67.532, -4.143) construction
  line L4321 (-67.532, -4.143) -> (-67.6833, -4.0812) construction
  line L4322 (-67.6833, -4.0812) -> (-67.8345, -4.0185) construction
  line L4323 (-67.8345, -4.0185) -> (-67.9856, -3.9548) construction
  line L4324 (-67.9856, -3.9548) -> (-68.1365, -3.8903) construction
  line L4325 (-68.1365, -3.8903) -> (-68.2872, -3.8249) construction
  line L4326 (-68.2872, -3.8249) -> (-68.4378, -3.7585) construction
  line L4327 (-68.4378, -3.7585) -> (-68.5882, -3.6913) construction
  line L4328 (-68.5882, -3.6913) -> (-68.7384, -3.6233) construction
  line L4329 (-68.7384, -3.6233) -> (-68.8885, -3.5543) construction
  line L4330 (-68.8885, -3.5543) -> (-69.0384, -3.4846) construction
  line L4331 (-69.0384, -3.4846) -> (-69.1881, -3.4139) construction
  line L4332 (-69.1881, -3.4139) -> (-69.3376, -3.3425) construction
  line L4333 (-69.3376, -3.3425) -> (-69.487, -3.2701) construction
  line L4334 (-69.487, -3.2701) -> (-69.6362, -3.197) construction
  line L4335 (-69.6362, -3.197) -> (-69.7852, -3.123) construction
  line L4336 (-69.7852, -3.123) -> (-69.934, -3.0482) construction
  line L4337 (-69.934, -3.0482) -> (-70.0826, -2.9726) construction
  line L4338 (-70.0826, -2.9726) -> (-70.2311, -2.8962) construction
  line L4339 (-70.2311, -2.8962) -> (-70.3793, -2.819) construction
  line L4340 (-70.3793, -2.819) -> (-70.5274, -2.741) construction
  line L4341 (-70.5274, -2.741) -> (-70.6752, -2.6622) construction
  line L4342 (-70.6752, -2.6622) -> (-70.8229, -2.5826) construction
  line L4343 (-70.8229, -2.5826) -> (-70.9703, -2.5023) construction
  line L4344 (-70.9703, -2.5023) -> (-71.1176, -2.4211) construction
  line L4345 (-71.1176, -2.4211) -> (-71.2352, -2.3556) construction
  line L4346 (-71.2352, -2.3556) -> (-71.3234, -2.3061) construction
  line L4347 (-71.3234, -2.3061) -> (-71.3821, -2.2729) construction
  line L4348 (-71.3821, -2.2729) -> (-71.4115, -2.2563) construction
  spline S58 degree 5 poles (-59.5542, -13.3622) (-59.5843, -13.369) (-59.6444, -13.3833) (-59.7338, -13.4071) (-59.8517, -13.4435) (-59.9973, -13.4951) (-60.1416, -13.5511) (-60.2852, -13.6099) (-60.4283, -13.6701) (-60.5711, -13.7313) (-60.7136, -13.7935) (-60.8557, -13.8571) (-60.9971, -13.9226) (-61.1379, -13.9902) (-61.2779, -14.06) (-61.4173, -14.1316) (-61.5561, -14.205) (-61.6944, -14.2797) (-61.8322, -14.3557) (-61.9697, -14.4327) (-62.1067, -14.5109) (-62.2432, -14.5904) (-62.3792, -14.6711) (-62.5148, -14.753) (-62.6498, -14.8363) (-62.7843, -14.9208) (-62.9184, -15.0064) (-63.052, -15.0932) (-63.1852, -15.181) (-63.318, -15.2698) (-63.4503, -15.3597) (-63.5821, -15.4506) (-63.7135, -15.5425) (-63.8445, -15.6354) (-63.975, -15.7293) (-64.105, -15.8242) (-64.2346, -15.92) (-64.3638, -16.0168) (-64.4926, -16.1146) (-64.6209, -16.2132) (-64.7488, -16.3127) (-64.8762, -16.4131) (-65.0032, -16.5144) (-65.1298, -16.6166) (-65.256, -16.7196) (-65.3817, -16.8235) (-65.507, -16.9283) (-65.6318, -17.0338) (-65.7562, -17.1402) (-65.8802, -17.2474) (-66.0038, -17.3555) (-66.1269, -17.4643) (-66.2497, -17.5739) (-66.3719, -17.6842) (-66.4938, -17.7954) (-66.6152, -17.9073) (-66.7362, -18.02) (-66.8568, -18.1335) (-66.9769, -18.2477) (-67.0966, -18.3626) (-67.2159, -18.4782) (-67.3347, -18.5946) (-67.4531, -18.7118) (-67.5711, -18.8296) (-67.6887, -18.9481) (-67.8058, -19.0674) (-67.9225, -19.1873) (-68.0388, -19.3079) (-68.1546, -19.4293) (-68.27, -19.5512) (-68.385, -19.6739) (-68.4767, -19.7726) (-68.5452, -19.8469) (-68.5908, -19.8966) (-68.6136, -19.9215) knots 0 0 0 0 0 0 0.01428571 0.02857143 0.04285714 0.05714286 0.07142857 0.08571429 0.1 0.11428571 0.12857143 0.14285714 0.15714286 0.17142857 0.18571429 0.2 0.21428571 0.22857143 0.24285714 0.25714286 0.27142857 0.28571429 0.3 0.31428571 0.32857143 0.34285714 0.35714286 0.37142857 0.38571429 0.4 0.41428571 0.42857143 0.44285714 0.45714286 0.47142857 0.48571429 0.5 0.51428571 0.52857143 0.54285714 0.55714286 0.57142857 0.58571429 0.6 0.61428571 0.62857143 0.64285714 0.65714286 0.67142857 0.68571429 0.7 0.71428571 0.72857143 0.74285714 0.75714286 0.77142857 0.78571429 0.8 0.81428571 0.82857143 0.84285714 0.85714286 0.87142857 0.88571429 0.9 0.91428571 0.92857143 0.94285714 0.95714286 0.97142857 0.98571429 1 1 1 1 1 1
  line L4349 (-59.5542, -13.3622) -> (-59.5843, -13.369) construction
  line L4350 (-59.5843, -13.369) -> (-59.6444, -13.3833) construction
  line L4351 (-59.6444, -13.3833) -> (-59.7338, -13.4071) construction
  line L4352 (-59.7338, -13.4071) -> (-59.8517, -13.4435) construction
  line L4353 (-59.8517, -13.4435) -> (-59.9973, -13.4951) construction
  line L4354 (-59.9973, -13.4951) -> (-60.1416, -13.5511) construction
  line L4355 (-60.1416, -13.5511) -> (-60.2852, -13.6099) construction
  line L4356 (-60.2852, -13.6099) -> (-60.4283, -13.6701) construction
  line L4357 (-60.4283, -13.6701) -> (-60.5711, -13.7313) construction
  line L4358 (-60.5711, -13.7313) -> (-60.7136, -13.7935) construction
  line L4359 (-60.7136, -13.7935) -> (-60.8557, -13.8571) construction
  line L4360 (-60.8557, -13.8571) -> (-60.9971, -13.9226) construction
  line L4361 (-60.9971, -13.9226) -> (-61.1379, -13.9902) construction
  line L4362 (-61.1379, -13.9902) -> (-61.2779, -14.06) construction
  line L4363 (-61.2779, -14.06) -> (-61.4173, -14.1316) construction
  line L4364 (-61.4173, -14.1316) -> (-61.5561, -14.205) construction
  line L4365 (-61.5561, -14.205) -> (-61.6944, -14.2797) construction
  line L4366 (-61.6944, -14.2797) -> (-61.8322, -14.3557) construction
  line L4367 (-61.8322, -14.3557) -> (-61.9697, -14.4327) construction
  line L4368 (-61.9697, -14.4327) -> (-62.1067, -14.5109) construction
  line L4369 (-62.1067, -14.5109) -> (-62.2432, -14.5904) construction
  line L4370 (-62.2432, -14.5904) -> (-62.3792, -14.6711) construction
  line L4371 (-62.3792, -14.6711) -> (-62.5148, -14.753) construction
  line L4372 (-62.5148, -14.753) -> (-62.6498, -14.8363) construction
  line L4373 (-62.6498, -14.8363) -> (-62.7843, -14.9208) construction
  line L4374 (-62.7843, -14.9208) -> (-62.9184, -15.0064) construction
  line L4375 (-62.9184, -15.0064) -> (-63.052, -15.0932) construction
  line L4376 (-63.052, -15.0932) -> (-63.1852, -15.181) construction
  line L4377 (-63.1852, -15.181) -> (-63.318, -15.2698) construction
  line L4378 (-63.318, -15.2698) -> (-63.4503, -15.3597) construction
  line L4379 (-63.4503, -15.3597) -> (-63.5821, -15.4506) construction
  line L4380 (-63.5821, -15.4506) -> (-63.7135, -15.5425) construction
  line L4381 (-63.7135, -15.5425) -> (-63.8445, -15.6354) construction
  line L4382 (-63.8445, -15.6354) -> (-63.975, -15.7293) construction
  line L4383 (-63.975, -15.7293) -> (-64.105, -15.8242) construction
  line L4384 (-64.105, -15.8242) -> (-64.2346, -15.92) construction
  line L4385 (-64.2346, -15.92) -> (-64.3638, -16.0168) construction
  line L4386 (-64.3638, -16.0168) -> (-64.4926, -16.1146) construction
  line L4387 (-64.4926, -16.1146) -> (-64.6209, -16.2132) construction
  line L4388 (-64.6209, -16.2132) -> (-64.7488, -16.3127) construction
  line L4389 (-64.7488, -16.3127) -> (-64.8762, -16.4131) construction
  line L4390 (-64.8762, -16.4131) -> (-65.0032, -16.5144) construction
  line L4391 (-65.0032, -16.5144) -> (-65.1298, -16.6166) construction
  line L4392 (-65.1298, -16.6166) -> (-65.256, -16.7196) construction
  line L4393 (-65.256, -16.7196) -> (-65.3817, -16.8235) construction
  line L4394 (-65.3817, -16.8235) -> (-65.507, -16.9283) construction
  line L4395 (-65.507, -16.9283) -> (-65.6318, -17.0338) construction
  line L4396 (-65.6318, -17.0338) -> (-65.7562, -17.1402) construction
  line L4397 (-65.7562, -17.1402) -> (-65.8802, -17.2474) construction
  line L4398 (-65.8802, -17.2474) -> (-66.0038, -17.3555) construction
  line L4399 (-66.0038, -17.3555) -> (-66.1269, -17.4643) construction
  line L4400 (-66.1269, -17.4643) -> (-66.2497, -17.5739) construction
  line L4401 (-66.2497, -17.5739) -> (-66.3719, -17.6842) construction
  line L4402 (-66.3719, -17.6842) -> (-66.4938, -17.7954) construction
  line L4403 (-66.4938, -17.7954) -> (-66.6152, -17.9073) construction
  line L4404 (-66.6152, -17.9073) -> (-66.7362, -18.02) construction
  line L4405 (-66.7362, -18.02) -> (-66.8568, -18.1335) construction
  line L4406 (-66.8568, -18.1335) -> (-66.9769, -18.2477) construction
  line L4407 (-66.9769, -18.2477) -> (-67.0966, -18.3626) construction
  line L4408 (-67.0966, -18.3626) -> (-67.2159, -18.4782) construction
  line L4409 (-67.2159, -18.4782) -> (-67.3347, -18.5946) construction
  line L4410 (-67.3347, -18.5946) -> (-67.4531, -18.7118) construction
  line L4411 (-67.4531, -18.7118) -> (-67.5711, -18.8296) construction
  line L4412 (-67.5711, -18.8296) -> (-67.6887, -18.9481) construction
  line L4413 (-67.6887, -18.9481) -> (-67.8058, -19.0674) construction
  line L4414 (-67.8058, -19.0674) -> (-67.9225, -19.1873) construction
  line L4415 (-67.9225, -19.1873) -> (-68.0388, -19.3079) construction
  line L4416 (-68.0388, -19.3079) -> (-68.1546, -19.4293) construction
  line L4417 (-68.1546, -19.4293) -> (-68.27, -19.5512) construction
  line L4418 (-68.27, -19.5512) -> (-68.385, -19.6739) construction
  line L4419 (-68.385, -19.6739) -> (-68.4767, -19.7726) construction
  line L4420 (-68.4767, -19.7726) -> (-68.5452, -19.8469) construction
  line L4421 (-68.5452, -19.8469) -> (-68.5908, -19.8966) construction
  line L4422 (-68.5908, -19.8966) -> (-68.6136, -19.9215) construction
  arc A109 (-10.6816, -56.435) -> (-13.005, -57.9623) centre (-11.0535, -58.4001) ccw
  arc A110 (-59.1442, 5.5428) -> (-56.9737, 7.2806) centre (-58.9575, 7.5341) ccw
  arc A111 (-51.1066, -30.2798) -> (-50.3721, -27.5982) centre (-52.1261, -28.5592) ccw
  arc A112 (-27.5982, -50.3721) -> (-30.2798, -51.1066) centre (-28.5592, -52.1261) ccw
  spline S59 degree 5 poles (-31.1115, -52.5103) (-31.1272, -52.5368) (-31.1594, -52.5895) (-31.2097, -52.6672) (-31.2807, -52.7681) (-31.3748, -52.8906) (-31.4727, -53.0106) (-31.5729, -53.1289) (-31.6744, -53.2464) (-31.7767, -53.3634) (-31.88, -53.4797) (-31.9844, -53.5951) (-32.0903, -53.7094) (-32.1981, -53.8224) (-32.3077, -53.934) (-32.419, -54.0444) (-32.5316, -54.1537) (-32.6455, -54.2622) (-32.7603, -54.3698) (-32.876, -54.4767) (-32.9927, -54.5828) (-33.1105, -54.6881) (-33.2292, -54.7926) (-33.3491, -54.8961) (-33.47, -54.9988) (-33.5919, -55.1007) (-33.7148, -55.2017) (-33.8386, -55.302) (-33.9633, -55.4015) (-34.0888, -55.5003) (-34.2151, -55.5984) (-34.3423, -55.6957) (-34.4703, -55.7923) (-34.5991, -55.8881) (-34.7288, -55.9832) (-34.8592, -56.0776) (-34.9905, -56.1712) (-35.1224, -56.2642) (-35.2552, -56.3564) (-35.3886, -56.448) (-35.5228, -56.5388) (-35.6577, -56.629) (-35.7933, -56.7185) (-35.9295, -56.8073) (-36.0665, -56.8955) (-36.2042, -56.9829) (-36.3425, -57.0697) (-36.4815, -57.1558) (-36.6211, -57.2413) (-36.7614, -57.3261) (-36.9023, -57.4102) (-37.0438, -57.4937) (-37.186, -57.5765) (-37.3288, -57.6587) (-37.4721, -57.7403) (-37.6161, -57.8212) (-37.7607, -57.9014) (-37.9058, -57.981) (-38.0515, -58.06) (-38.1978, -58.1383) (-38.3447, -58.216) (-38.4921, -58.2931) (-38.6401, -58.3695) (-38.7886, -58.4453) (-38.9377, -58.5205) (-39.0873, -58.595) (-39.2374, -58.669) (-39.3881, -58.7423) (-39.5393, -58.8149) (-39.6909, -58.887) (-39.8431, -58.9584) (-39.9653, -59.0151) (-40.0572, -59.0573) (-40.1185, -59.0853) (-40.1492, -59.0993) knots 0 0 0 0 0 0 0.01428571 0.02857143 0.04285714 0.05714286 0.07142857 0.08571429 0.1 0.11428571 0.12857143 0.14285714 0.15714286 0.17142857 0.18571429 0.2 0.21428571 0.22857143 0.24285714 0.25714286 0.27142857 0.28571429 0.3 0.31428571 0.32857143 0.34285714 0.35714286 0.37142857 0.38571429 0.4 0.41428571 0.42857143 0.44285714 0.45714286 0.47142857 0.48571429 0.5 0.51428571 0.52857143 0.54285714 0.55714286 0.57142857 0.58571429 0.6 0.61428571 0.62857143 0.64285714 0.65714286 0.67142857 0.68571429 0.7 0.71428571 0.72857143 0.74285714 0.75714286 0.77142857 0.78571429 0.8 0.81428571 0.82857143 0.84285714 0.85714286 0.87142857 0.88571429 0.9 0.91428571 0.92857143 0.94285714 0.95714286 0.97142857 0.98571429 1 1 1 1 1 1
  line L4423 (-31.1115, -52.5103) -> (-31.1272, -52.5368) construction
  line L4424 (-31.1272, -52.5368) -> (-31.1594, -52.5895) construction
  line L4425 (-31.1594, -52.5895) -> (-31.2097, -52.6672) construction
  line L4426 (-31.2097, -52.6672) -> (-31.2807, -52.7681) construction
  line L4427 (-31.2807, -52.7681) -> (-31.3748, -52.8906) construction
  line L4428 (-31.3748, -52.8906) -> (-31.4727, -53.0106) construction
  line L4429 (-31.4727, -53.0106) -> (-31.5729, -53.1289) construction
  line L4430 (-31.5729, -53.1289) -> (-31.6744, -53.2464) construction
  line L4431 (-31.6744, -53.2464) -> (-31.7767, -53.3634) construction
  line L4432 (-31.7767, -53.3634) -> (-31.88, -53.4797) construction
  line L4433 (-31.88, -53.4797) -> (-31.9844, -53.5951) construction
  line L4434 (-31.9844, -53.5951) -> (-32.0903, -53.7094) construction
  line L4435 (-32.0903, -53.7094) -> (-32.1981, -53.8224) construction
  line L4436 (-32.1981, -53.8224) -> (-32.3077, -53.934) construction
  line L4437 (-32.3077, -53.934) -> (-32.419, -54.0444) construction
  line L4438 (-32.419, -54.0444) -> (-32.5316, -54.1537) construction
  line L4439 (-32.5316, -54.1537) -> (-32.6455, -54.2622) construction
  line L4440 (-32.6455, -54.2622) -> (-32.7603, -54.3698) construction
  line L4441 (-32.7603, -54.3698) -> (-32.876, -54.4767) construction
  line L4442 (-32.876, -54.4767) -> (-32.9927, -54.5828) construction
  line L4443 (-32.9927, -54.5828) -> (-33.1105, -54.6881) construction
  line L4444 (-33.1105, -54.6881) -> (-33.2292, -54.7926) construction
  line L4445 (-33.2292, -54.7926) -> (-33.3491, -54.8961) construction
  line L4446 (-33.3491, -54.8961) -> (-33.47, -54.9988) construction
  line L4447 (-33.47, -54.9988) -> (-33.5919, -55.1007) construction
  line L4448 (-33.5919, -55.1007) -> (-33.7148, -55.2017) construction
  line L4449 (-33.7148, -55.2017) -> (-33.8386, -55.302) construction
  line L4450 (-33.8386, -55.302) -> (-33.9633, -55.4015) construction